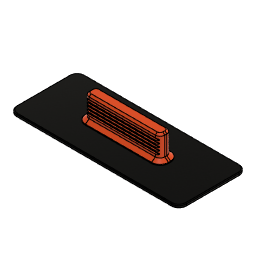
Stínítko displeje v7 (Autodesk Fusion 360 design; units mm, degrees)
Autodesk Fusion 360 part; units mm, degrees
sketch "Sketch1" plane through (0, 0, 0) normal (0, 0, 1) x (1, 0, 0)
  line L0 (41, -15) -> (-41, -15)
  line L1 (-42, -14) -> (-42, 14)
  line L2 (-41, 15) -> (41, 15)
  line L3 (42, 14) -> (42, -14)
  line L4 (42, -15) -> (-42, 15) construction
  line L5 (-42, -15) -> (42, 15) construction
  arc A0 (-41, 15) -> (-42, 14) centre (-41, 14) ccw
  arc A1 (42, 14) -> (41, 15) centre (41, 14) ccw
  arc A2 (41, -15) -> (42, -14) centre (41, -14) ccw
  arc A3 (-42, -14) -> (-41, -15) centre (-41, -14) ccw
  line L6 (41, -18) -> (-41, -18)
  arc A4 (-45, -14) -> (-41, -18) centre (-41, -14) ccw
  line L7 (-45, -14) -> (-45, 14)
  arc A5 (-41, 18) -> (-45, 14) centre (-41, 14) ccw
  line L8 (-41, 18) -> (41, 18)
  arc A6 (45, 14) -> (41, 18) centre (41, 14) ccw
  line L9 (45, 14) -> (45, -14)
  arc A7 (41, -18) -> (45, -14) centre (41, -14) ccw
  circle A8 centre (-15, 0) radius 2.05
  circle A9 centre (-15, 0) radius 3
  line L10 (0, 1.75) -> (0, 22.5)
  circle A10 centre (15, 0) radius 2.05
  circle A11 centre (15, 0) radius 3
  line L11 (-20.05, 3.05) -> (20.05, 3.05)
  line L12 (20.05, 3.05) -> (20.05, -3.05)
  line L13 (20.05, -3.05) -> (-20.05, -3.05)
  line L14 (-20.05, -3.05) -> (-20.05, 3.05)
  line L15 (-20.05, 3.05) -> (20.05, -3.05) construction
  line L16 (20.05, 3.05) -> (-20.05, -3.05) construction
  circle A12 centre (-15, 0) radius 2.5
  circle A13 centre (-15, 0) radius 1.95
  circle A14 centre (15, 0) radius 1.95
  circle A15 centre (15, 0) radius 2.5
  dimension "d1" = 84
  dimension "d2" = 30
  dimension "d3" = -3
  dimension "d4" = 1
  dimension "d12" = 4.1
  dimension "d13" = 6
  dimension "d14" = 15
  dimension "d16" = 1
  dimension "d17" = 3
  dimension "d18" = -0.5
  dimension "d19" = -0.1
  constraint horizontal L0
  constraint perpendicular L0 L1
  constraint parallel L0 L2
  constraint parallel L1 L3
  constraint coincident L4 origin
  constraint coincident L5 origin
  constraint coincident L4.end L1
  constraint coincident L4.end L2
  constraint tangent L1 A0
  constraint tangent L2 A0
  constraint coincident L5.end L2
  constraint coincident L5.end L3
  constraint tangent L2 A1
  constraint tangent L3 A1
  constraint equal A0 A1
  constraint coincident L4.start L3
  constraint coincident L4.start L0
  constraint tangent L3 A2
  constraint tangent L0 A2
  constraint equal A0 A2
  constraint coincident L5.start L0
  constraint coincident L5.start L1
  constraint tangent L0 A3
  constraint tangent L1 A3
  constraint equal A0 A3
  constraint concentric A8 A9
  constraint horizontal origin A8.centre
  constraint symmetric A8 L10 A10
  constraint symmetric A9 L10 A11
  constraint horizontal L11
  constraint perpendicular L11 L12
  constraint parallel L11 L13
  constraint parallel L12 L14
  constraint coincident L15 origin
  constraint coincident L16 origin
  constraint symmetric L10 A12 A15
  constraint symmetric L10 A13 A14
  measures "d1" distance of L4.end L5.end
  measures "d2" distance of L5.start L4.end
  measures "d4" radius of A0
  measures "d12" diameter of A8
  measures "d13" diameter of A9
  measures "d14" distance of origin A8.centre
  measures "d16" distance of A8 L11
  measures "d17" distance of A8 L14
extrude "Extrude1" add sketch "Sketch1" against normal blind 1.5 contours L0 L1 L2 L3 A0 A1 A2 A3 | A8 | A9 | A10 | A11 | L11 L12 L13 L14 | A12 | A13 | A14 | A15 makes body 1
extrude "Extrude2" add sketch "Sketch1" along normal blind 1.5 contours L0 L1 L2 L3 A0 A1 A2 A3 | L6 A4 L7 A5 L8 A6 L9 A7 | A8 | A9 | A10 | A11 | L11 L12 L13 L14 | A12 | A13 | A14 | A15 bodies 1
chamfer "Chamfer1" distance 0.4 angle 45 2 faces at (13.6667, -6, 1.5) (-13.6667, -5, -1.5) on bodies 1
chamfer "Chamfer1" distance 0.1 angle 45 8 edges at (0, -15, 0) (-41.7071, -14.7071, 0) (-42, 0, 0) (-41.7071, 14.7071, 0) (0, 15, 0) (41.7071, 14.7071, 0) (42, 0, 0) (41.7071, -14.7071, 0) on bodies 1
chamfer "Chamfer1" distance 0.2 angle 45 8 edges at (0, -18, 0) (-43.8284, -16.8284, 0) (-45, 0, 0) (-43.8284, 16.8284, 0) (0, 18, 0) (43.8284, 16.8284, 0) (45, 0, 0) (43.8284, -16.8284, 0) on bodies 1
extrude "Extrude3" cut sketch "Sketch1" along normal up to surface (1.5 mm away) contours A8 | A10 | A13 | A14 bodies 1
extrude "Extrude4" cut sketch "Sketch1" against normal up to surface (1.5 mm away) contours A8 | A9 | A10 | A11 | A12 | A13 | A14 | A15 bodies 1
chamfer "Chamfer2" distance 0.5 angle 45 2 edges at (-16.9113, 0.7413, 1.5) (13.0887, 0.7413, 1.5) on bodies 1
chamfer "Chamfer2" distance 0.2 angle 45 3 edges at (-17.797, -1.0848, -1.5) (12.203, -1.0848, -1.5) (12.203, -1.0848, 0) on bodies 1
extrude "Extrude5" add sketch "Sketch1" along normal blind 13 from surface at 1.5 separate body contours A8 | A9 | A10 | A11 | L11 L12 L13 L14 | A12 | A13 | A14 | A15 makes body 2
extrude "Extrude6" add sketch "Sketch1" along normal blind 10 from surface at 0.2 contours A13 | A14 bodies 2
fillet "Fillet1" radius 2.5 4 edges at (20.05, 3.05, 8) (20.05, -3.05, 8) (-20.05, 3.05, 8) (-20.05, -3.05, 8) on bodies 2
chamfer "Chamfer5" distance 1 angle 45 8 edges at (0, 3.05, 14.5) (-19.3178, 2.3178, 14.5) (-20.05, 0, 14.5) (-19.3178, -2.3178, 14.5) (0, -3.05, 14.5) (19.3178, -2.3178, 14.5) (20.05, 0, 14.5) (19.3178, 2.3178, 14.5) on bodies 2
sketch "Sketch3" plane through (-20.05, 0, 0) normal (-1, 0, 0) x (0, -1, 0)
  line L0 (0.55, 1.5) -> (0.55, 13.5)
  line L1 (0.55, 13.5) -> (-0.55, 13.5)
  line L2 (-0.55, 13.5) -> (-0.55, 1.5)
  line L3 (-3.45, 12.5) -> (-2.45, 12)
  line L4 (-2.45, 12) -> (-2.45, 11.5)
  line L5 (-2.45, 11.5) -> (-3.45, 11)
  line L6 (-0.55, 13.5) -> (-3.05, 13.5)
  line L7 (-3.05, 13.5) -> (-3.05, 1.5)
  line L8 (-3.45, 10.9) -> (-2.45, 10.4)
  line L9 (-2.45, 10.4) -> (-2.45, 9.9)
  line L10 (-2.45, 9.9) -> (-3.45, 9.4)
  line L11 (-3.45, 9.3) -> (-2.45, 8.8)
  line L12 (-2.45, 8.8) -> (-2.45, 8.3)
  line L13 (-2.45, 8.3) -> (-3.45, 7.8)
  line L14 (-3.45, 7.7) -> (-2.45, 7.2)
  line L15 (-2.45, 7.2) -> (-2.45, 6.7)
  line L16 (-2.45, 6.7) -> (-3.45, 6.2)
  line L17 (-3.45, 6.1) -> (-2.45, 5.6)
  line L18 (-2.45, 5.6) -> (-2.45, 5.1)
  line L19 (-2.45, 5.1) -> (-3.45, 4.6)
  line L20 (0, 1.75) -> (0, 22.5)
  line L21 (3.45, 7.7) -> (2.45, 7.2)
  line L22 (2.45, 10.4) -> (2.45, 9.9)
  line L23 (2.45, 5.6) -> (2.45, 5.1)
  line L24 (2.45, 7.2) -> (2.45, 6.7)
  line L25 (2.45, 6.7) -> (3.45, 6.2)
  line L26 (2.45, 11.5) -> (3.45, 11)
  line L27 (2.45, 12) -> (2.45, 11.5)
  line L28 (2.45, 5.1) -> (3.45, 4.6)
  line L29 (3.45, 9.3) -> (2.45, 8.8)
  line L30 (2.45, 9.9) -> (3.45, 9.4)
  line L31 (2.45, 8.3) -> (3.45, 7.8)
  line L32 (3.45, 12.5) -> (2.45, 12)
  line L33 (2.45, 8.8) -> (2.45, 8.3)
  line L34 (3.45, 10.9) -> (2.45, 10.4)
  line L35 (3.45, 6.1) -> (2.45, 5.6)
  line L36 (3.45, 4.6) -> (3.45, 12.5)
  line L37 (-3.45, 12.5) -> (-3.45, 4.6)
  line L38 (-0.55, 1.5) -> (0.55, 1.5)
  point P0 (-0.55, 14.5)
  dimension "d47" = 0.5
  dimension "d48" = 0.5
  dimension "d49" = 0.5
  dimension "d50" = 1
  dimension "d51" = 1
  dimension "d53" = 0.6
  dimension "d56" = 0
  dimension "d57" = -1.6
  constraint vertical L4
  constraint vertical L3.start L5.end
  constraint symmetric L3.start L20 L32.start
  constraint symmetric L3.end L20 L27.start
  constraint symmetric L4.end L20 L26.start
  constraint symmetric L5.end L20 L26.end
  constraint symmetric L8.start L20 L34.start
  constraint symmetric L8.end L20 L22.start
  constraint symmetric L9.end L20 L22.end
  constraint symmetric L10.end L20 L30.end
  constraint symmetric L11.start L20 L29.start
  constraint symmetric L11.end L20 L29.end
  constraint symmetric L12.end L20 L31.start
  constraint symmetric L13.end L20 L31.end
  constraint symmetric L14.start L20 L21.start
  constraint symmetric L14.end L20 L21.end
  constraint symmetric L15.end L20 L24.end
  constraint symmetric L16.end L20 L25.end
  constraint symmetric L17.start L20 L35.start
  constraint symmetric L17.end L20 L23.start
  constraint symmetric L18.end L20 L23.end
  constraint symmetric L19.end L20 L28.end
  measures "d47" distance of L3.end L4.end
  measures "d48" vertical distance of L3.start L3.end
  measures "d49" vertical distance of L4.end L5.end
  measures "d50" distance of L4 L5.end
  measures "d51" distance of L3.start L6
  measures "d53" distance of L4.end L7
extrude "Extrude10" cut sketch "Sketch3" against normal up to surface (40.1 mm away) contours L3 L5 L7 L37 | L3 L4 L5 L7 | L7 L8 L10 L37 | L7 L8 L9 L10 | L7 L11 L13 L37 | L7 L11 L12 L13 | L7 L14 L16 L37 | L7 L14 L15 L16 | L7 L17 L19 L37 | L7 L17 L18 L19 | L21 L24 L25 L36 | L22 L30 L34 L36 | L23 L28 L35 L36 | L26 L27 L32 L36 | L29 L31 L33 L36 bodies 2
chamfer "Chamfer7" distance 0.5 angle 45 2 edges at (-16.818, -0.7052, 1.5) (13.182, -0.7052, 1.5) on bodies 2
hole "Hole1" at (-15, 0, 0.2) direction (0, 0, 1) diameter 2.4 depth 12 tip angle 180 countersink diameter 3 countersink angle 90 bodies 2
hole "Hole2" at (15, -0.0284, 0.2) direction (0, 0, 1) diameter 2.4 depth 12 tip angle 180 countersink diameter 3 countersink angle 90 bodies 2
chamfer "Chamfer8" distance 0.3 angle 45 2 edges at (-13.8812, 0.4339, 12.2) (16.1188, 0.4055, 12.2) on bodies 2
sketch "Sketch4" plane through (0, 0, 1.5) normal (0, 0, -1) x (1, 0, 0)
  circle A0 centre (-15, 0) radius 2.45
  arc A1 (-17.55, 3.05) -> (-20.05, 0.55) centre (-17.55, 0.55) ccw
  line L0 (-20.05, 0.55) -> (-20.05, -0.55)
  arc A2 (-20.05, -0.55) -> (-17.55, -3.05) centre (-17.55, -0.55) ccw
  line L1 (-17.55, -3.05) -> (17.55, -3.05)
  arc A3 (17.55, -3.05) -> (20.05, -0.55) centre (17.55, -0.55) ccw
  line L2 (20.05, -0.55) -> (20.05, 0.55)
  arc A4 (20.05, 0.55) -> (17.55, 3.05) centre (17.55, 0.55) ccw
  line L3 (17.55, 3.05) -> (-17.55, 3.05)
  circle A5 centre (15, 0) radius 2.45
  line L4 (-22.05, 0.55) -> (-22.05, -0.55)
  arc A6 (-22.05, -0.55) -> (-17.55, -5.05) centre (-17.55, -0.55) ccw
  line L5 (-17.55, -5.05) -> (17.55, -5.05)
  arc A7 (17.55, -5.05) -> (22.05, -0.55) centre (17.55, -0.55) ccw
  line L6 (22.05, -0.55) -> (22.05, 0.55)
  arc A8 (22.05, 0.55) -> (17.55, 5.05) centre (17.55, 0.55) ccw
  line L7 (17.55, 5.05) -> (-17.55, 5.05)
  arc A9 (-17.55, 5.05) -> (-22.05, 0.55) centre (-17.55, 0.55) ccw
  dimension "d75" = 2
extrude "Extrude11" add sketch "Sketch4" against normal blind 2 contours L4 A6 L5 A7 L6 A8 L7 A9 bodies 2
chamfer "Chamfer9" distance 2 distance2 1.5 8 edges at (0, -5.05, 3.5) (20.732, -3.732, 3.5) (22.05, 0, 3.5) (20.732, 3.732, 3.5) (0, 5.05, 3.5) (-20.732, 3.732, 3.5) (-22.05, 0, 3.5) (-20.732, -3.732, 3.5) measured on face at (5.85, -3.7167, 3.5) measured on face at (5.85, -3.7167, 3.5) measured on face at (5.85, -3.7167, 3.5) measured on face at (5.85, -3.7167, 3.5) measured on face at (5.85, -3.7167, 3.5) measured on face at (5.85, -3.7167, 3.5) measured on face at (5.85, -3.7167, 3.5) measured on face at (5.85, -3.7167, 3.5) on bodies 2
named bodies: "Plate", "Handle"
